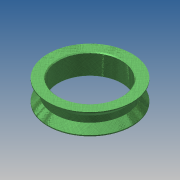
# Autodesk Inventor part: Seilrolle
Saved by Autodesk Inventor 2015 SP1 (Build 190203100, 203)
## iProperties
Created: 2015-02-20
Part Number: Seilrolle
Material: ABS-Kunststoff
Document SubType Name: Modeling
Designer: Marc
Mass: 0.437978 g
Surface Area: 8.13749 cm^2
Volume: 0.413186 cm^3
Density: 1.06 g/cm^3
Appearance: Gehont - dunkelgrau
Author: Marc
Autodesk Inventor part; units mm, degrees
ref_plane "YZ Plane" through (0, 0, 0) normal (1, 0, 0) x (0, 1, 0)
ref_plane "XZ Plane" through (0, 0, 0) normal (0, 1, 0) x (-1, 0, 0)
ref_plane "XY Plane" through (0, 0, 0) normal (0, 0, 1) x (1, 0, 0)
sketch "Skizze1" plane through (0, 0, 0) normal (0, 0, 1) x (1, 0, 0)
  line L0 (-14, 0) -> (14, 0) projected
  line L1 (0, -14) -> (0, 14) projected
  circle A0 centre (0, 0) radius 7.5
  circle A1 centre (0, 0) radius 10
  dimension "d0" = 15
  dimension "d1" = 20
  constraints: 2 centre point, 2 coincident
  measures "d0" diameter of A0
  measures "d1" diameter of A1
extrude "Extrusion1" add sketch "Skizze1" along normal mid plane 5 contours A0 L1 A1 L0 | L0 A1 L1 A0 | A0 L0 A1 L1 | L1 A1 L0 A0
sketch "Skizze2" plane through (0, 0, 0) normal (0, 0, 1) x (1, 0, 0)
  circle A0 centre (0, 0) radius 7.5 projected
  circle A1 centre (0, 0) radius 10 projected
  circle A2 centre (0, 0) radius 7.5 projected
  circle A3 centre (0, 0) radius 10 projected
  line L0 (-14, 0) -> (14, 0) projected
  line L1 (0, -14) -> (0, 14) projected
  circle A4 centre (0, 0) radius 8.5
  dimension "d4" = 17
  constraints: 1 centre point, 1 coincident
  measures "d4" diameter of A4
extrude "Extrusion2" cut sketch "Skizze2" along normal mid plane 1.5 contours A4 L1 A1 L0 | L0 A1 L1 A4 | A4 L0 A1 L1 | L1 A1 L0 A4
chamfer "Fase1" distance 1.5 angle 45 2 edges at (-10, 0, 0.75) (-10, 0, -0.75)
chamfer "Fase2" distance 0.2 angle 45 1 edges at (-7.5, 0, 2.5)
chamfer "Fase3" distance 0.2 angle 45 1 edges at (-7.5, 0, -2.5)
